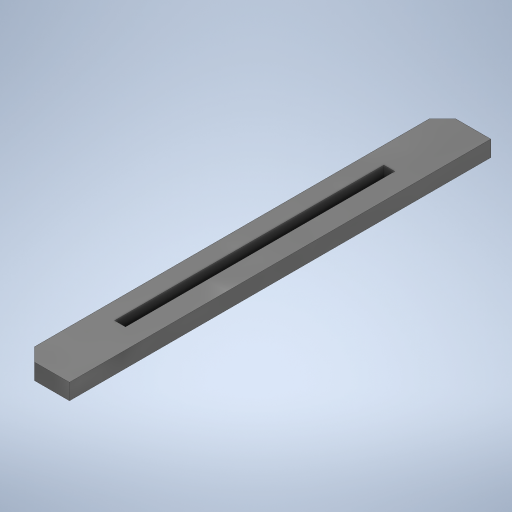
# Autodesk Inventor part: insert spacer - v2
Saved by Autodesk Inventor 2024 (Build 280153000, 153)
## iProperties
Created: 2023-09-15
Part Number: insert spacer - v2
Material: Generic
Document SubType Name: Modeling
Designer: cfang
Density: 1 g/cm^3
Appearance: Default
Author: cfang
Autodesk Inventor part; units mm, degrees
ref_plane "YZ Plane" through (0, 0, 0) normal (1, 0, 0) x (0, 1, 0)
ref_plane "XZ Plane" through (0, 0, 0) normal (0, 1, 0) x (-1, 0, 0)
ref_plane "XY Plane" through (0, 0, 0) normal (0, 0, 1) x (1, 0, 0)
sketch "Sketch1" plane through (0, 0, 0) normal (0, 1, 0) x (-1, 0, 0)
  line L0 (-0.955, -7.9) -> (0.855, -7.9)
  line L1 (0.855, -7.9) -> (0.855, 7.9)
  line L2 (0.855, 7.9) -> (-0.955, 7.9)
  line L3 (-0.955, 7.9) -> (-0.955, -7.9)
  point P0 (0, 0)
  dimension "d0" = 15.8
  dimension "d7" = 0.855
  dimension "d8" = 0.955
  constraints: 8 end point, 2 parallel, 1 horizontal, 1 perpendicular
  measures "d0" distance of L0.end L1.end
  measures "d7" distance from line of point (0, 0) L1
  measures "d8" distance from line of point (0, 0) L3
extrude "Extrusion1" add sketch "Sketch1" along normal blind 0.6
sketch "Sketch2" plane through (0, 0.6, 0) normal (0, 1, 0) x (1, 0, 0)
  line L0 (0.205, 5.05) -> (-0.205, 5.05)
  line L1 (-0.205, 5.05) -> (-0.205, -5.05)
  line L2 (-0.205, -5.05) -> (0.205, -5.05)
  line L3 (0.205, -5.05) -> (0.205, 5.05)
  line L4 (0.205, 5.05) -> (-0.205, -5.05) construction
  line L5 (-0.205, 5.05) -> (0.205, -5.05) construction
  point P0 (0, 0)
  dimension "d3" = 0.41
  dimension "d4" = 10.1
  constraints: 12 end point, 2 midpoint, 2 parallel, 1 horizontal, 1 perpendicular
  measures "d3" distance of L1.end L2.end
  measures "d4" distance of L0.end L1.end
extrude "Extrusion2" cut sketch "Sketch2" against normal through all
sketch "Sketch3" plane through (0, 0.6, 0) normal (0, 1, 0) x (1, 0, 0)
  line L0 (-0.855, 7.9) -> (-0.855, -7.9) projected
  line L1 (-0.855, -7.4) -> (-0.355, -7.9)
  line L2 (-0.855, -7.9) -> (0.955, -7.9) projected
  line L3 (0.955, 7.9) -> (-0.855, 7.9) projected
  line L4 (-0.855, 7.4) -> (-0.355, 7.9)
  point P0 (0, 0)
  dimension "d9" = 0.5
  dimension "d10" = 0.5
  dimension "d11" = 0.5
  dimension "d12" = 0.5
  constraints: 4 end point, 4 point on line
  measures "d9" distance of L1.start L0.end
  measures "d10" distance of L1.end L0.end
  measures "d11" distance of L4.start L0.start
  measures "d12" distance of L4.end L0.start
extrude "Extrusion3" cut sketch "Sketch3" against normal through all
body "Solid1"
